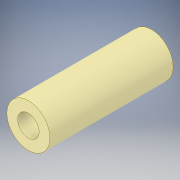
# Autodesk Inventor part: CLB_082_ScissorsPulleySpacerShorter
Saved by Autodesk Inventor 2018.3 (Build 223284000, 284)
## iProperties
Created: 2020-02-21
Part Number: CLB_082_ScissorsPulleySpacerShorter
Material: Nylon 6/6
Document SubType Name: Modeling
Designer: 22perngrac
Density: 1.13 g/cm^3
Appearance: Nylon 6
Author: 22perngrac
Autodesk Inventor part; units mm, degrees
ref_plane "YZ Plane" through (0, 0, 0) normal (1, 0, 0) x (0, 1, 0)
ref_plane "XZ Plane" through (0, 0, 0) normal (0, 1, 0) x (-1, 0, 0)
ref_plane "XY Plane" through (0, 0, 0) normal (0, 0, 1) x (1, 0, 0)
sketch "Sketch1" plane through (0, 0, 0) normal (0, 0, 1) x (1, 0, 0)
  circle A0 centre (0, 0) radius 6.35
  dimension "d0" = 12.7
  constraints: 1 centre point, 1 coincident
  measures "d0" diameter of A0
extrude "Extrusion1" add sketch "Sketch1" along normal blind 36.322
sketch "Sketch2" plane through (0, 0, 36.322) normal (0, 0, 1) x (1, 0, 0)
  point P0 (0, 0)
  point P1 (0, 0)
  constraints: 1 coincident
hole "Hole1" at (0, 0, 36.322) direction (0, 0, -1) diameter 6.35 end through all
body "Solid1"
